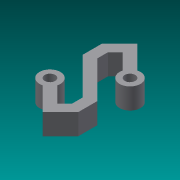
# Autodesk Inventor part: Sawaiz Logo
Saved by Autodesk Inventor 2015 (Build 190159000, 159)
## iProperties
Created: 2015-06-22
Part Number: Sawaiz Logo
Material: Generic
Document SubType Name: Modeling
Designer: Sawaiz Syed
Density: 1 g/cm^3
Appearance: Default
Author: Sawaiz Syed
Autodesk Inventor part; units mm, degrees
ref_plane "YZ Plane" through (0, 0, 0) normal (1, 0, 0) x (0, 1, 0)
ref_plane "XZ Plane" through (0, 0, 0) normal (0, 1, 0) x (-1, 0, 0)
ref_plane "XY Plane" through (0, 0, 0) normal (0, 0, 1) x (1, 0, 0)
sketch "Sketch1" plane through (0, 0, 0) normal (0, 0, 1) x (1, 0, 0)
  circle A0 centre (0, 0) radius 2.5
  circle A1 centre (0, 0) radius 5
  line L0 (-1.7678, -1.7678) -> (-12.3744, 8.8388)
  line L1 (-12.3744, 8.8388) -> (-15.9099, 5.3033)
  line L2 (-15.9099, 5.3033) -> (-15.9099, 0.3033)
  line L3 (-15.9099, 0.3033) -> (1.7678, -17.3744)
  line L4 (1.7678, -17.3744) -> (1.7678, -26.5165)
  line L5 (1.7678, -26.5165) -> (-6.7678, -35.052)
  line L6 (-6.7678, -35.052) -> (-20.9099, -20.9099)
  line L7 (1.7678, 1.7678) -> (-12.3744, 15.9099)
  line L8 (-12.3744, 15.9099) -> (-20.9099, 7.3744)
  line L9 (-20.9099, 7.3744) -> (-20.9099, -1.7678)
  line L10 (-20.9099, -1.7678) -> (-3.2322, -19.4454)
  line L11 (-3.2322, -19.4454) -> (-3.2322, -24.4454)
  line L12 (-3.2322, -24.4454) -> (-6.7678, -27.981)
  line L13 (-6.7678, -27.981) -> (-17.3744, -17.3744)
  line L14 (-17.3744, -17.3744) -> (-20.9099, -20.9099)
  line L15 (-1.7678, -1.7678) -> (1.7678, 1.7678)
  circle A2 centre (-19.1421, -19.1421) radius 2.5
  circle A3 centre (-19.1421, -19.1421) radius 5
  dimension "d0" = 5
  dimension "d1" = 10
  dimension "d3" = 90
  dimension "d4" = 135
  dimension "d5" = 135
  dimension "d6" = 135
  dimension "d7" = 135
  dimension "d8" = 90
  dimension "d9" = 5
  dimension "d12" = 10
  dimension "d13" = 15
  dimension "d14" = 15
  dimension "d15" = 5
  dimension "d16" = 5
  dimension "d17" = 5
  dimension "d18" = 5
  dimension "d20" = 20
  dimension "d21" = 20
  dimension "d22" = 5
  dimension "d23" = 5
  dimension "d24" = 5
  constraints: 32 end point, 4 centre point, 4 parallel, 3 coincident, 3 tangent, 2 collinear, 2 perpendicular, 2 point on circle, 1 midpoint, 1 vertical
  measures "d0" diameter of A0
  measures "d1" diameter of A1
  measures "d3" angle of L1 L0
  measures "d4" angle of L2 L1
  measures "d5" angle of L3 L2
  measures "d6" angle of L3 L4
  measures "d7" angle of L4 L5
  measures "d8" angle of L5 L6
  measures "d9" distance of L13.end L6.end
  measures "d12" diameter of A3
  measures "d13" distance of L0.start L0.end
  measures "d14" distance of L12.end L13.end
  measures "d15" distance of L0.end L1.end
  measures "d16" distance of L1.end L2.end
  measures "d17" distance of L11.end L12.end
  measures "d18" distance of L10.end L11.end
  measures "d20" distance of L7.start L7.end
  measures "d21" distance of L5.end L6.end
  measures "d22" distance between parallel lines of L10 L3
  measures "d23" distance between parallel lines of L2 L9
  measures "d24" distance between parallel lines of L4 L11
extrude "Extrusion2" add sketch "Sketch1" along normal blind 10 contours A0 L7 A1 L0 | A0 L0 A1 L7 | A1 L0 L1 L2 L3 L4 L5 L6 A3 L13 L12 L11 L10 L9 L8 L7 | A3 L6 A2 L13 | L13 A2 L6 A3 | A2 L14 picked at (-18.68, -20.1685)
sketch "Sketch2" plane through (0, 0, 10) normal (0, 0, 1) x (1, 0, 0)
  line L0 (-1.2941, 4.8296) -> (-12.3744, 15.9099) projected
  line L1 (-12.3744, 15.9099) -> (-20.9099, 7.3744) projected
  line L2 (-20.9099, 7.3744) -> (-20.9099, -1.7678) projected
  line L3 (-20.9099, -1.7678) -> (-3.2322, -19.4454) projected
  line L4 (-3.2322, -19.4454) -> (-3.2322, -24.4454) projected
  line L5 (-3.2322, -24.4454) -> (-6.7678, -27.981) projected
  line L6 (-6.7678, -27.981) -> (-14.3125, -20.4362) projected
  arc A0 (-14.3125, -20.4362) -> (-17.848, -23.9718) centre (-19.1421, -19.1421) ccw projected
  line L7 (-17.848, -23.9718) -> (-6.7678, -35.052) projected
  line L8 (-6.7678, -35.052) -> (1.7678, -26.5165) projected
  line L9 (1.7678, -26.5165) -> (1.7678, -17.3744) projected
  line L10 (1.7678, -17.3744) -> (-15.9099, 0.3033) projected
  line L11 (-15.9099, 0.3033) -> (-15.9099, 5.3033) projected
  line L12 (-15.9099, 5.3033) -> (-12.3744, 8.8388) projected
  line L13 (-12.3744, 8.8388) -> (-4.8296, 1.2941) projected
  arc A1 (-4.8296, 1.2941) -> (-1.2941, 4.8296) centre (0, 0) ccw projected
  line L14 (-20.9099, -20.9099) -> (-17.3744, -17.3744) projected
  arc A2 (-17.3744, -17.3744) -> (-20.9099, -20.9099) centre (-19.1421, -19.1421) ccw projected
  circle A3 centre (0, 0) radius 2.5 projected
  circle A4 centre (-19.1421, -19.1421) radius 2.5
  constraints: 1 centre point, 1 coincident, 1 concentric
extrude "Extrusion3" cut sketch "Sketch2" against normal blind 10 contours L14 A4
equation "\"d1\" = 2 * d0"
equation "\"d9\" = d0"
equation "\"d12\" = d1"
equation "\"d13\" = 3 * d0"
equation "\"d14\" = d13"
equation "\"d15\" = d0"
equation "\"d17\" = d15"
equation "\"d18\" = d16"
body "Solid2"
